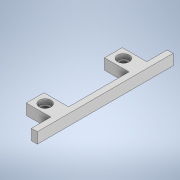
# Autodesk Inventor part: support_2
Saved by Autodesk Inventor 2020 (Build 240168000, 168)
## iProperties
Created: 2019-11-28
Part Number: support_2
Material: Generic
Document SubType Name: Modeling
Designer: sl65b
Density: 1 g/cm^3
Appearance: Default
Author: sl65b
Autodesk Inventor part; units mm, degrees
ref_plane "YZ Plane" through (0, 0, 0) normal (1, 0, 0) x (0, 1, 0)
ref_plane "XZ Plane" through (0, 0, 0) normal (0, 1, 0) x (-1, 0, 0)
ref_plane "XY Plane" through (0, 0, 0) normal (0, 0, 1) x (1, 0, 0)
sketch "Sketch1" plane through (0, 0, 0) normal (0, 1, 0) x (-1, 0, 0)
  line L0 (-9.22, 34.5) -> (9.22, 34.5)
  line L1 (9.22, 34.5) -> (9.22, -34.5)
  line L2 (9.22, -34.5) -> (-9.22, -34.5)
  line L3 (-9.22, -34.5) -> (-9.22, 34.5)
  line L4 (-9.22, 34.5) -> (9.22, -34.5) construction
  line L5 (9.22, 34.5) -> (-9.22, -34.5) construction
  point P0 (0, 0)
  dimension "d0" = 18.44
  dimension "d1" = 69
  constraints: 12 end point, 2 midpoint, 2 parallel, 1 horizontal, 1 perpendicular
  measures "d0" distance of L1.end L2.end
  measures "d1" distance of L0.end L1.end
extrude "Extrusion1" add sketch "Sketch1" along normal blind 5.5
sketch "Sketch4" plane through (0, 5.5, 0) normal (0, 1, 0) x (1, 0, 0)
  circle A0 centre (-1.16, 19.65) radius 2.4879
  line L0 (-9.22, 34.5) -> (-9.22, -34.5) projected
  line L1 (-9.22, -34.5) -> (9.22, -34.5) projected
  point P0 (0, 0)
  dimension "d6" = 8.06
  dimension "d7" = 54.15
  constraints: 1 centre point
  measures "d6" distance from line of L0 A0.centre
  measures "d7" distance from line of L1 A0.centre
hole "Hole1" at (-1.16, 5.5, -19.65) direction (0, -1, 0) diameter 3.5 depth 10.5 tip angle 118 counterbore diameter 6 counterbore depth 2.3
sketch "Sketch5" plane through (0, 5.5, 0) normal (0, 1, 0) x (1, 0, 0)
  circle A0 centre (-1.16, -20.15) radius 2.6607
  line L0 (-9.22, 34.5) -> (-9.22, -34.5) projected
  line L1 (-9.22, -34.5) -> (9.22, -34.5) projected
  point P0 (0, 0)
  dimension "d15" = 8.06
  dimension "d16" = 14.35
  constraints: 1 centre point
  measures "d15" distance from line of L0 A0.centre
  measures "d16" distance from line of L1 A0.centre
hole "Hole2" at (-1.16, 5.5, 20.15) direction (0, -1, 0) diameter 3.5 depth 10.5 tip angle 118 counterbore diameter 6 counterbore depth 2.3
sketch "Sketch6" plane through (0, 5.5, 0) normal (0, 1, 0) x (1, 0, 0)
  line L0 (-9.22, -34.5) -> (9.22, -34.5) projected
  line L1 (-9.22, 34.5) -> (-9.22, -34.5) projected
  line L2 (6.22, -34.5) -> (-9.22, -34.5)
  line L3 (-9.22, -34.5) -> (-9.22, 34.5)
  line L4 (-9.22, 34.5) -> (6.22, 34.5)
  line L5 (6.22, 34.5) -> (6.22, -34.5)
  line L6 (9.22, -34.5) -> (9.22, 34.5) projected
  line L7 (6.22, -15.65) -> (-6.2399, -15.65)
  line L8 (-6.2399, -15.65) -> (-6.2399, -24.65)
  line L9 (-6.2399, -24.65) -> (6.22, -24.65)
  line L10 (6.22, 15.15) -> (-6.2399, 15.15)
  line L11 (-6.2399, 15.15) -> (-6.2399, 24.15)
  line L12 (-6.2399, 24.15) -> (6.22, 24.15)
  circle A0 centre (-1.16, -20.15) radius 3 projected
  circle A1 centre (-1.16, 19.65) radius 3 projected
  point P0 (0, 0)
  dimension "d24" = 3
  dimension "d25" = 9
  dimension "d26" = 9
  dimension "d27" = 4.5
  dimension "d28" = 4.5
  constraints: 20 end point, 7 point on line, 4 perpendicular, 3 parallel, 2 horizontal
  measures "d24" distance between parallel lines of L6 L5
  measures "d25" distance of L7.end L8.end
  measures "d26" distance of L10.end L11.end
  measures "d27" distance from line of L9 A0.centre
  measures "d28" distance from line of L10 A1.centre
extrude "Extrusion2" cut sketch "Sketch6" against normal blind 9 contours L1 L4 L5 L12 L11 L10 L7 L8 L9 L0
body "Solid1"
